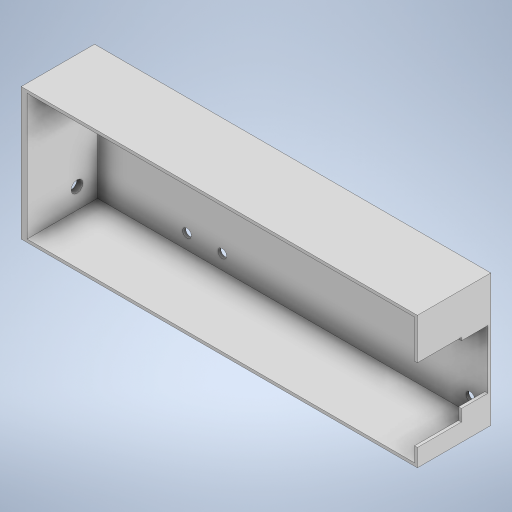
# Autodesk Inventor part: arduino mould
Saved by Autodesk Inventor 2023 (Build 270158000, 158)
## iProperties
Created: 2023-05-03
Part Number: arduino mould
Material: Generic
Document SubType Name: Modeling
Designer: gmami
Density: 1 g/cm^3
Appearance: Default
Author: gmami
Autodesk Inventor part; units mm, degrees
ref_plane "YZ Plane" through (0, 0, 0) normal (1, 0, 0) x (0, 1, 0)
ref_plane "XZ Plane" through (0, 0, 0) normal (0, 1, 0) x (-1, 0, 0)
ref_plane "XY Plane" through (0, 0, 0) normal (0, 0, 1) x (1, 0, 0)
sketch "Sketch1" plane through (0, 0, 0) normal (0, 0, 1) x (1, 0, 0)
  line L0 (-119.142, 1.6299) -> (13.858, 1.6299)
  line L1 (14.858, 0.6299) -> (14.858, -42.3701)
  line L2 (13.858, -43.3701) -> (-119.142, -43.3701)
  line L3 (-120.142, -42.3701) -> (-120.142, 0.6299)
  arc A0 (-119.142, 1.6299) -> (-120.142, 0.6299) centre (-119.142, 0.6299) ccw
  arc A1 (-120.142, -42.3701) -> (-119.142, -43.3701) centre (-119.142, -42.3701) ccw
  arc A2 (13.858, -43.3701) -> (14.858, -42.3701) centre (13.858, -42.3701) ccw
  arc A3 (14.858, 0.6299) -> (13.858, 1.6299) centre (13.858, 0.6299) ccw
  circle A4 centre (8.858, -4.3701) radius 1.5
  circle A5 centre (-87.642, -37.3701) radius 1.5
  circle A6 centre (-75.642, -37.3701) radius 1.5
  circle A7 centre (8.858, -37.3701) radius 1.5
  circle A8 centre (-87.642, -4.3701) radius 1.5
  circle A9 centre (-75.642, -4.3701) radius 1.5
  point P0 (0, 0)
  point P1 (-120.142, 1.6299)
  point P2 (14.858, 1.6299)
  dimension "d0" = 135
  dimension "d2" = 1
  dimension "d3" = 1
  dimension "d7" = 3
  dimension "d8" = 6
  dimension "d9" = 6
  dimension "d10" = 3
  dimension "d11" = 3
  dimension "d14" = 3
  dimension "d15" = 6
  dimension "d16" = 6
  dimension "d17" = 6
  dimension "d18" = 6
  dimension "d19" = 12
  dimension "d20" = 32.5
  dimension "d21" = 3
  dimension "d22" = 3
  dimension "d23" = 6
  dimension "d24" = 6
  dimension "d25" = 32.5
  dimension "d26" = 12
  constraints: 10 centre point, 8 end point, 8 point on circle, 8 tangent, 4 point on line, 2 equal radius, 2 parallel, 1 horizontal, 1 perpendicular
  measures "d0" distance of point (-120.142, 1.63) point (14.858, 1.63)
  measures "d2" radius of A0
  measures "d3" radius of A1
  measures "d7" diameter of A4
  measures "d8" distance from line of L0 A4.centre
  measures "d9" distance from line of L1 A4.centre
  measures "d10" diameter of A5
  measures "d11" diameter of A6
  measures "d14" diameter of A7
  measures "d15" distance from line of L2 A7.centre
  measures "d16" distance from line of L1 A7.centre
  measures "d17" distance from line of L2 A6.centre
  measures "d18" distance from line of L2 A5.centre
  measures "d19" distance of A6.centre A5.centre
  measures "d20" distance from line of L3 A5.centre
  measures "d21" diameter of A8
  measures "d22" diameter of A9
  measures "d23" distance from line of L0 A9.centre
  measures "d24" distance from line of L0 A8.centre
  measures "d25" distance from line of A8.centre L3
  measures "d26" distance of A9.centre A8.centre
extrude "Extrusion1" add sketch "Sketch1" along normal blind 1
sketch "Sketch2" plane through (14.858, -42.3701, 0) normal (1, 0, 0) x (0, 0, -1)
  line L0 (0, 44) -> (-1, 44) projected
  line L1 (-25, -1) -> (0, -1)
  line L2 (0, -1) -> (0, 44)
  line L3 (0, 44) -> (-25, 44)
  line L4 (-25, 44) -> (-25, -1)
  line L5 (0, 0) -> (0, -1) projected
  line L6 (0, -1) -> (-10, -1)
  line L7 (-10, -1) -> (-10, 44)
  line L8 (-10, 44) -> (0, 44)
  line L9 (0, 44) -> (0, -1)
  line L10 (0, -1) -> (-1, -1)
  line L11 (-1, -1) -> (-1, 44)
  line L12 (-1, 44) -> (0, 44)
  line L13 (0, 44) -> (0, -1)
  line L14 (-1, 0) -> (-1, 43) projected
  line L15 (-10, 9) -> (-1, 9)
  line L16 (-1, 9) -> (-1, 29)
  line L17 (-1, 29) -> (-10, 29)
  line L18 (-10, 29) -> (-10, 9)
  line L19 (-25, 5) -> (-10, 5)
  line L20 (-10, 5) -> (-10, 30)
  line L21 (-10, 30) -> (-25, 30)
  line L22 (-25, 30) -> (-25, 5)
  point P0 (0, 42.3701)
  point P1 (-1, 9)
  dimension "d29" = 25
  dimension "d30" = 10
  dimension "d31" = 10
  dimension "d32" = 20
  dimension "d33" = 6
  dimension "d34" = 25
  constraints: 40 end point, 10 parallel, 5 horizontal, 5 perpendicular, 5 point on line
  measures "d29" distance of L1.start L1.end
  measures "d30" distance between parallel lines of L2 L7
  measures "d31" distance between parallel lines of L15 L6
  measures "d32" distance between parallel lines of L17 L15
  measures "d33" distance between parallel lines of L1 L19
  measures "d34" distance between parallel lines of L21 L19
extrude "Extrusion2" add sketch "Sketch2" against normal blind 1 contours L11 L17 L7 L3 | L7 L21 L4 L3 | L1 L7 L15 L11 | L1 L4 L19 L7
sketch "Sketch3" plane through (-119.142, -43.3701, 0) normal (0, -1, 0) x (1, 0, 0)
  line L0 (0, 0) -> (-1, 0) projected
  line L1 (134, 25) -> (134, 10) projected
  line L2 (-1, 0) -> (134, 0)
  line L3 (134, 0) -> (134, 25)
  line L4 (134, 25) -> (-1, 25)
  line L5 (-1, 25) -> (-1, 0)
  point P0 (119.142, 0)
  constraints: 8 end point, 2 parallel, 1 horizontal, 1 perpendicular
extrude "Extrusion3" add sketch "Sketch3" against normal blind 1
sketch "Sketch4" plane through (-119.142, 1.6299, 0) normal (0, 1, 0) x (1, 0, 0)
  line L0 (134, -25) -> (134, -10) projected
  line L1 (-1, 0) -> (-1, -1) projected
  line L2 (134, -25) -> (-1, -25)
  line L3 (-1, -25) -> (-1, 0)
  line L4 (-1, 0) -> (134, 0)
  line L5 (134, 0) -> (134, -25)
  point P0 (119.142, 0)
  constraints: 8 end point, 2 parallel, 1 horizontal, 1 perpendicular
sketch "Sketch5" plane through (-120.142, -43.3701, 0) normal (-1, 0, 0) x (0, 0, 1)
  line L0 (25, 45) -> (1, 45) projected
  line L1 (0, 44) -> (0, 0) projected
  line L2 (25, 45) -> (0, 45)
  line L3 (0, 45) -> (0, 0)
  line L4 (0, 0) -> (25, 0)
  line L5 (25, 0) -> (25, 45)
  circle A0 centre (8, 33) radius 2
  circle A1 centre (8, 8) radius 2
  point P0 (0, 43.3701)
  point P1 (1, 45)
  dimension "d39" = 25
  dimension "d40" = 12
  dimension "d42" = 8
  dimension "d47" = 4
  dimension "d48" = 4
  dimension "d49" = 8
  constraints: 8 end point, 2 centre point, 2 parallel, 1 horizontal, 1 perpendicular
  measures "d39" distance of A1.centre A0.centre
  measures "d40" distance from line of L0 A0.centre
  measures "d42" distance from line of L4 A1.centre
  measures "d47" diameter of A0
  measures "d48" diameter of A1
  measures "d49" distance from line of L1 A0.centre
extrude "Extrusion4" add sketch "Sketch5" against normal blind 2
extrude "Extrusion5" add sketch "Sketch4" against normal blind 1
body "Solid1"
